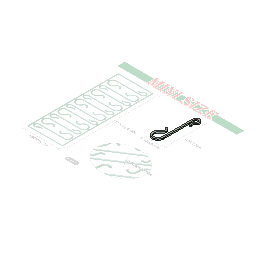
Christmas Ornament Hooks (Autodesk Fusion 360 design; units mm, degrees)
Autodesk Fusion 360 part; units mm, degrees
sketch "Sketch1" plane through (0, 0, 0) normal (0, 0, 1) x (1, 0, 0) in component "Carabiner Style"
  line L0 (0, 0) -> (15, 0) construction
  line L1 (15, 0) -> (15, 40) construction
  line L2 (15, 40) -> (0, 40) construction
  line L3 (0, 40) -> (0, 0) construction
  circle A0 centre (12.5, 37.5) radius 2.5
  circle A1 centre (5.9624, 5.9624) radius 5.9624
  line L4 (10.1208, 38.2677) -> (0.2881, 7.7932)
  line L5 (11.8745, 5.1899) -> (14.9883, 37.2584)
  dimension "d1" = 40
  dimension "d2" = 15
  dimension "d3" = 5
  constraint horizontal L0
  constraint vertical L1
  constraint horizontal L2
  constraint vertical L3
  constraint coincident L0.start L3.end
  constraint tangent L2 A0
  constraint tangent L1 A0
  constraint tangent L0 A1
  constraint tangent L3 A1
  constraint coincident A0 L4.start
  constraint coincident A1 L4.end
  constraint tangent A0 L4
  constraint tangent A1 L4
  constraint coincident A1 L5.start
  constraint coincident A0 L5.end
  constraint tangent A0 L5
  measures "d1" distance of L0.start L2.end
  measures "d2" distance of L0.start L0.end
  measures "d3" diameter of A0
sketch "Sketch1 (2)" plane through (0, 0, 0) normal (0, 0, 1) x (1, 0, 0) in component "Hook Style"
  spline S0 degree 5 poles (-1.9882, 10.2998) (-1.75, 10.205) (-1.2978, 10.0036) (-0.6915, 9.6658) (-0.0276, 9.1441) (0.5609, 8.3788) (0.9085, 7.5176) (1.018, 6.5999) (0.8969, 5.6834) (0.5554, 4.8792) (0.0265, 4.2117) (-0.6398, 3.6431) (-1.3819, 3.103) (-2.1317, 2.5133) (-2.8194, 1.8161) (-3.3789, 0.9995) (-3.7525, 0.0872) (-3.8951, -0.8724) (-3.7797, -1.8167) (-3.4017, -2.6789) (-2.785, -3.3994) (-1.9815, -3.9322) (-1.0588, -4.2454) (-0.0931, -4.3246) (0.8411, -4.1737) (1.6791, -3.8184) (2.3753, -3.3073) (2.9028, -2.7015) (3.2549, -2.0651) (3.4451, -1.4557) (3.5104, -0.9134) (3.5066, -0.5474) (3.4944, -0.3135) (3.4853, -0.1754) (3.4805, -0.1108) knots 0 0 0 0 0 0 0.033333 0.066667 0.1 0.133333 0.166667 0.2 0.233333 0.266667 0.3 0.333333 0.366667 0.4 0.433333 0.466667 0.5 0.533333 0.566667 0.6 0.633333 0.666667 0.7 0.733333 0.766667 0.8 0.833333 0.866667 0.9 0.933333 0.966667 1 1 1 1 1 1
  line L0 (3.4805, -0.1108) -> (3.5386, 29.9156)
  spline S1 degree 5 poles (3.5386, 29.9156) (3.5454, 30.0433) (3.5691, 30.2942) (3.6357, 30.6573) (3.7862, 31.1147) (4.0768, 31.6403) (4.4671, 32.1154) (4.9506, 32.5318) (5.5158, 32.876) (6.1441, 33.1277) (6.8108, 33.2624) (7.4874, 33.2572) (8.1436, 33.0957) (8.7488, 32.7732) (9.2744, 32.302) (9.696, 31.7166) (9.9942, 31.0648) (10.1564, 30.3987) (10.1782, 29.7665) (10.0648, 29.2035) (9.8332, 28.7222) (9.5118, 28.3093) (9.1354, 27.9374) (8.7412, 27.5744) (8.3647, 27.1921) (8.0348, 26.7782) (7.7721, 26.3376) (7.5912, 25.8851) (7.5016, 25.4404) (7.5088, 25.0215) (7.6155, 24.6396) (7.7814, 24.3677) (7.951, 24.1834) (8.0842, 24.0693) (8.1558, 24.0144) knots 0 0 0 0 0 0 0.033333 0.066667 0.1 0.133333 0.166667 0.2 0.233333 0.266667 0.3 0.333333 0.366667 0.4 0.433333 0.466667 0.5 0.533333 0.566667 0.6 0.633333 0.666667 0.7 0.733333 0.766667 0.8 0.833333 0.866667 0.9 0.933333 0.966667 1 1 1 1 1 1
  line L1 (1.1874, 7.6859) -> (0.637, 4.3838)
  line L2 (3.5745, -1.3767) -> (3.3866, 1.1552)
  spline S2 degree 3 poles (-2.5799, 8.8133) (-1.6533, 8.4444) (-1.1684, 8.017) (-0.9116, 7.5998) (-0.694, 7.2461) (-0.6099, 6.8396) (-0.6484, 6.4331) (-0.6819, 6.0794) (-0.7891, 5.8089) (-0.9947, 5.5395) (-1.2322, 5.2282) (-1.6857, 4.8767) (-2.3252, 4.3852) (-3.1138, 3.7792) (-4.1101, 2.909) (-4.7407, 1.7355) (-5.3204, 0.6567) (-5.5929, -0.67) (-5.325, -1.9401) (-5.0758, -3.1213) (-4.3455, -4.1999) (-3.3703, -4.8901) (-2.1134, -5.7798) (-0.4918, -6.0554) (0.9352, -5.7421) (2.3063, -5.4411) (3.4517, -4.6033) (4.1411, -3.6515) (4.7451, -2.8176) (5.0079, -1.8951) (5.0764, -1.1967) (5.126, -0.6905) (5.0994, -0.3283) (5.0807, -0.0554) knots 0 0 0 0 0.096555 0.096555 0.096555 0.178378 0.178378 0.178378 0.249569 0.249569 0.249569 0.33182 0.33182 0.33182 0.433243 0.433243 0.433243 0.526475 0.526475 0.526475 0.613175 0.613175 0.613175 0.724926 0.724926 0.724926 0.832295 0.832295 0.832295 0.926367 0.926367 0.926367 0.994548 0.994548 0.994548 0.994548
  line L3 (5.0807, -0.0554) -> (5.1385, 29.8664)
  spline S3 degree 3 poles (5.1385, 29.8664) (5.171, 30.3407) (5.3133, 30.6486) (5.6198, 30.9671) (5.9638, 31.3246) (6.5799, 31.6226) (7.0528, 31.6404) (7.4576, 31.6557) (7.7512, 31.541) (8.0505, 31.2129) (8.32, 30.9173) (8.5213, 30.4194) (8.5478, 30.0887) (8.567, 29.8485) (8.5338, 29.7371) (8.4701, 29.6166) (8.3975, 29.4794) (8.2041, 29.2659) (7.8444, 28.923) (7.373, 28.4736) (6.7199, 27.7992) (6.3311, 26.988) (5.9683, 26.2312) (5.7841, 25.3355) (6.0246, 24.4381) (6.2061, 23.7607) (6.6504, 23.1523) (7.1824, 22.7446) knots 0.003152 0.003152 0.003152 0.003152 0.131534 0.131534 0.131534 0.275585 0.275585 0.275585 0.398889 0.398889 0.398889 0.509937 0.509937 0.509937 0.590585 0.590585 0.590585 0.682461 0.682461 0.682461 0.802858 0.802858 0.802858 0.9152 0.9152 0.9152 1 1 1 1
  line L4 (8.1558, 24.0144) -> (7.1824, 22.7446)
  line L5 (-2.5799, 8.8133) -> (-1.9882, 10.2998)
  point P0 (0.9122, 6.0349)
  point P1 (-2.1147, 2.4881)
  point P2 (-3.5518, -2.251)
  point P3 (0.7288, -4.1467)
  point P4 (3.3665, -1.6552)
  point P5 (5.1581, 32.6411)
  point P6 (8.722, 32.7411)
  point P7 (10.0876, 29.4103)
  point P8 (8.5554, 27.3785)
  point P9 (7.5229, 25.4134)
  dimension "d4" = 1.6
  constraint midpoint P0 L1
  constraint midpoint S0.end L2
extrude "Extrude1" add sketch "Sketch1 (2)" along normal blind 1.2 in component "Hook Style"
fillet "Fillet1" radius 0.8 4 edges at (7.1824, 22.7446, 0.6) (8.1558, 24.0144, 0.6) (-2.5799, 8.8133, 0.6) (-1.9882, 10.2998, 0.6) in component "Hook Style"
component "Carabiner Style" placed x (1, 0, 0) y (0, 1, 0) z (0, 0, 1) at (0, 0, 0)
component "Hook Style" placed x (1, 0, 0) y (0, 1, 0) z (0, 0, 1) at (0, 0, 0)
named bodies: "Hook Style"
